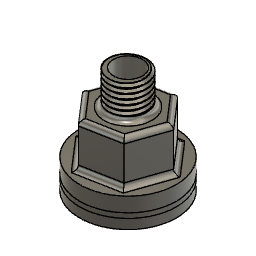
Dræn på tank P3 v1 (Autodesk Fusion 360 design; units mm, degrees)
Autodesk Fusion 360 part; units mm, degrees
sketch "Sketch1" plane through (0, 0, 0) normal (0, 1, 0) x (1, 0, 0)
  circle A0 centre (0, 0) radius 12.5
  circle A1 centre (0, 0) radius 25
  dimension "d1" = 25
  dimension "d2" = 50
  constraint coincident A0.centre A1.centre
  constraint concentric A0 A1
  measures "d1" diameter of A0
  measures "d2" diameter of A1
extrude "Extrude1" add sketch "Sketch1" along normal blind 7.5 contours A0 | A1 makes body 1
sketch "Sketch2" plane through (0, 7.5, 0) normal (0, 1, 0) x (-1, 0, 0)
  circle A0 centre (0, 0) radius 25
  circle A1 centre (0, 0) radius 12.5
  dimension "d5" = 25
  constraint concentric A0 A1
  measures "d5" diameter of A1
extrude "Extrude2" add sketch "Sketch2" along normal blind 22.5 contours A1 bodies 1
sketch "Sketch3" plane through (0, 30, 0) normal (0, 1, 0) x (-1, 0, 0)
  circle A0 centre (0, 0) radius 12.5
  circle A1 centre (0, 0) radius 8.75
  dimension "d8" = 17.5
  constraint coincident A0.centre A1.centre
  measures "d8" diameter of A1
extrude "Extrude3" cut sketch "Sketch3" against normal blind 64 contours A1 bodies 1
thread "Thread1" "ISO Metric profile 25.0 M25x2 6g" major diameter 24.822 minor diameter 22.5289 pitch 2 angle 60 modelled right hand crest width 0.2818 on face at (-12.4845, 22.5, -0.6231) crest through (-12.411, 7, 0) on bodies 1
sketch "Sketch4" plane through (0, 30, 0) normal (0, 1, 0) x (-1, 0, 0)
  spline S0 degree 3 poles (9.172, 6.5392) (8.3735, 7.7838) (7.3376, 8.8588) (4.8917, 10.5716) (3.4995, 11.1843) (0.532, 11.8526) (-1.0168, 11.8916) (-4.0709, 11.374) (-5.5449, 10.8121) (-7.78, 9.4193) (-8.6094, 8.7352) (-10.0779, 7.1597) (-10.7081, 6.273) (-11.215, 5.3157) knots 0 0 0 0 0.443615 0.443615 0.895426 0.895426 1.35543 1.35543 1.823624 1.823624 2.144258 2.144258 2.468655 2.468655 2.468655 2.468655
  arc A0 (-11.215, 5.3157) -> (-11.215, -5.3157) centre (0, 0) ccw
  spline S1 degree 3 poles (-11.215, -5.3157) (-10.4658, -6.7305) (-9.4497, -7.9867) (-7.011, -10.0173) (-5.6188, -10.7802) (-2.6451, -11.7162) (-1.0955, -11.8902) (1.9552, -11.6318) (3.4278, -11.2123) (5.6738, -10.0602) (6.5063, -9.4849) (7.9889, -8.1389) (8.6348, -7.3766) (9.172, -6.5392) knots 0 0 0 0 0.48029 0.48029 0.952378 0.952378 1.41626 1.41626 1.871933 1.871933 2.174689 2.174689 2.473673 2.473673 2.473673 2.473673
  arc A1 (9.172, -6.5392) -> (9.172, 6.5392) centre (0, 0) ccw
  circle A2 centre (0, 0) radius 8.75
  circle A3 centre (0, 0) radius 12.5
  circle A4 centre (0, 0) radius 17.5
  dimension "d13" = 25
  dimension "d14" = 35
  constraint coincident A0.centre A1.centre
  constraint concentric A3 A4
  measures "d13" diameter of A3
  measures "d14" diameter of A4
extrude "Extrude4" add sketch "Sketch4" against normal up to surface (22.5 mm away) separate body contours A4 makes body 2
sketch "Sketch5" plane through (0, 7.5, 0) normal (0, -1, 0) x (1, 0, 0)
  circle A0 centre (0, 0) radius 12.5
  circle A1 centre (0, 0) radius 17.5
  circle A2 centre (0, 0) radius 25
  dimension "d17" = 50
  constraint concentric A0 A2
  measures "d17" diameter of A2
extrude "Extrude5" add sketch "Sketch5" against normal blind 7.5 contours A2 bodies 2
sketch "Sketch6" plane through (0, 30, 0) normal (0, 1, 0) x (-1, 0, 0)
  circle A0 centre (0, 0) radius 17.5
  line L0 (-19.8504, -3.781) -> (-6.6507, -19.0814)
  line L1 (-6.6507, -19.0814) -> (13.1996, -15.3004)
  line L2 (13.1996, -15.3004) -> (19.8504, 3.781)
  line L3 (19.8504, 3.781) -> (6.6507, 19.0814)
  line L4 (6.6507, 19.0814) -> (-13.1996, 15.3004)
  line L5 (-13.1996, 15.3004) -> (-19.8504, -3.781)
  circle A1 centre (0, 0) radius 12.5
  constraint coincident A0.centre A1.centre
  constraint tangent A0 L5
extrude "Extrude6" add sketch "Sketch6" against normal up to surface (15 mm away) contours A0 L2 L3 | A0 L3 L4 | A0 L1 L2 | A0 L4 L5 | A0 L0 L1 | A0 L0 L5 bodies 2
sketch "Sketch7" plane through (0, 30, 0) normal (0, 1, 0) x (-1, 0, 0)
  circle A0 centre (0, 0) radius 12.5
  line L0 (-6.6507, -19.0814) -> (13.1996, -15.3004)
  line L1 (13.1996, -15.3004) -> (19.8504, 3.781)
  line L2 (19.8504, 3.781) -> (6.6507, 19.0814)
  line L3 (6.6507, 19.0814) -> (-13.1996, 15.3004)
  line L4 (-13.1996, 15.3004) -> (-19.8504, -3.781)
  line L5 (-19.8504, -3.781) -> (-6.6507, -19.0814)
extrude "Extrude7" add sketch "Sketch7" along normal blind 7.5 contours A0 | L0 L1 L2 L3 L4 L5 bodies 2
sketch "Sketch8" plane through (0, 37.5, 0) normal (0, 1, 0) x (-1, 0, 0)
  line L0 (-19.8504, -3.781) -> (-6.6507, -19.0814)
  line L1 (-6.6507, -19.0814) -> (13.1996, -15.3004)
  line L2 (13.1996, -15.3004) -> (19.8504, 3.781)
  line L3 (19.8504, 3.781) -> (6.6507, 19.0814)
  line L4 (6.6507, 19.0814) -> (-13.1996, 15.3004)
  line L5 (-13.1996, 15.3004) -> (-19.8504, -3.781)
  circle A0 centre (0, 0) radius 10
  circle A1 centre (0, 0) radius 7.5
  dimension "d26" = 20
  dimension "d27" = 15
  constraint coincident A0.centre A1.centre
  constraint concentric A0 A1
  measures "d26" diameter of A0
  measures "d27" diameter of A1
extrude "Extrude8" add sketch "Sketch8" along normal blind 17.5 contours A0 bodies 2
fillet "Fillet1" radius 2.5 1 edges at (9.3233, 37.5, 3.6162) on bodies 2
fillet "Fillet2" radius 2.5 6 edges at (-16.525, 37.5, -5.7597) (-13.2505, 37.5, 11.4312) (3.2745, 37.5, 17.1909) (16.525, 37.5, 5.7597) (13.2505, 37.5, -11.4312) (-3.2745, 37.5, -17.1909) on bodies 2
fillet "Fillet3" radius 2.5 6 edges at (3.2745, 15, 17.1909) (-13.2505, 15, 11.4312) (-16.525, 15, -5.7597) (-3.2745, 15, -17.1909) (13.2505, 15, -11.4312) (16.525, 15, 5.7597) on bodies 2
thread "Thread3" "ISO Metric profile 20.0 M20x2.5 6g" major diameter 19.7905 minor diameter 16.938 pitch 2.5 angle 60 modelled right hand crest width 0.36 on face at (-9.9503, 50, -0.9957) crest through (-9.8953, 39.375, 0) on bodies 2
extrude "Extrude9" cut 1 faces at (-1.8326, 37.5, 1.7004) along direction (0, -1, 0) blind 5000 on bodies 2 bodies 2
extrude "Extrude10" add 1 faces at (20.6937, 7.5, -1.863) along direction (0, -1, 0) blind 2.5 on bodies 2 bodies 2
chamfer "Chamfer1" distance 4 angle 45 1 edges at (6.9925, 30, -2.7121) on bodies 2
thread "Thread4" "ISO Metric profile 25.0 M25x2 6H" major diameter 25.2565 minor diameter 23.0224 pitch 2 angle 60 modelled right hand crest width 0.5434 on face at (-12.4845, 13.3333, -0.6231) crest through (-11.5112, 29.5, 0) on bodies 2
